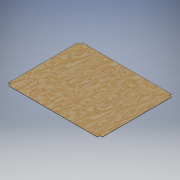
# Autodesk Inventor part: cart plywood
Saved by Autodesk Inventor 2016 SP2 (Build 200236200, 236)
## iProperties
Created: 2018-02-13
Part Number: cart plywood
Material: Generic
Document SubType Name: Modeling
Designer: CAD
Density: 1 g/cm^3
Appearance: Plywood - Weathered
Author: CAD
Autodesk Inventor part; units mm, degrees
ref_plane "YZ Plane" through (0, 0, 0) normal (1, 0, 0) x (0, 1, 0)
ref_plane "XZ Plane" through (0, 0, 0) normal (0, 1, 0) x (-1, 0, 0)
ref_plane "XY Plane" through (0, 0, 0) normal (0, 0, 1) x (1, 0, 0)
sketch "Sketch1" plane through (0, 0, 0) normal (0, 1, 0) x (-1, 0, 0)
  line L0 (508, 355.6) -> (508, -355.6)
  line L1 (508, -355.6) -> (482.6, -355.6)
  line L2 (482.6, -355.6) -> (482.6, -381)
  line L3 (482.6, -381) -> (-431.8, -381)
  line L4 (-431.8, -381) -> (-431.8, -355.6)
  line L5 (-431.8, -355.6) -> (-457.2, -355.6)
  line L6 (-457.2, -355.6) -> (-457.2, 355.6)
  line L7 (-457.2, 355.6) -> (-431.8, 355.6)
  line L8 (-431.8, 355.6) -> (-431.8, 381)
  line L9 (-431.8, 381) -> (482.6, 381)
  line L10 (482.6, 381) -> (482.6, 355.6)
  line L11 (482.6, 355.6) -> (508, 355.6)
  point P0 (0, 0)
  dimension "d0" = 711.2
  dimension "d1" = 25.4
  dimension "d2" = 25.4
  dimension "d4" = 25.4
  dimension "d5" = 25.4
  dimension "d6" = 711.2
  dimension "d7" = 25.4
  dimension "d8" = 25.4
  dimension "d10" = 25.4
  dimension "d11" = 508
  dimension "d12" = 381
  dimension "d15" = 914.4
  constraints: 24 end point, 6 point on line, 4 perpendicular, 1 vertical
  measures "d0" distance of L0.start L0.end
  measures "d1" distance of L0.end L1.end
  measures "d2" distance of L1.end L2.end
  measures "d4" distance of L3.end L4.end
  measures "d5" distance of L4.end L5.end
  measures "d6" distance of L5.end L6.end
  measures "d7" distance of L6.end L7.end
  measures "d8" distance of L7.end L8.end
  measures "d10" distance of L9.end L10.end
  measures "d11" distance from line of point (0, 0) L0
  measures "d12" distance from line of L9 point (0, 0)
  measures "d15" distance of L8.end L9.end
extrude "Extrusion1" add sketch "Sketch1" along normal blind 3.175
body "Solid1"
